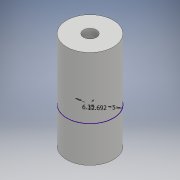
# Autodesk Inventor part: springHolder_final
Saved by Autodesk Inventor 2018 (Build 220112000, 112)
## iProperties
Created: 2017-11-09
Part Number: springHolder_final
Material: Generic
Document SubType Name: Modeling
Designer: Payal Jindal
Density: 1 g/cm^3
Appearance: Default
Author: Payal Jindal
Autodesk Inventor part; units mm, degrees
ref_plane "YZ Plane" through (0, 0, 0) normal (1, 0, 0) x (0, 1, 0)
ref_plane "XZ Plane" through (0, 0, 0) normal (0, 1, 0) x (-1, 0, 0)
ref_plane "XY Plane" through (0, 0, 0) normal (0, 0, 1) x (1, 0, 0)
sketch "Sketch1" plane through (0, 0, 0) normal (0, 0, 1) x (1, 0, 0)
  circle A0 centre (0, 0) radius 6.346
  circle A1 centre (0, 0) radius 11.346
  circle A2 centre (0, 0) radius 3.175
  dimension "d0" = 12.692
  dimension "d1" = 5
  dimension "d2" = 6.35
  constraints: 3 centre point, 3 coincident
  measures "d0" diameter of A0
  measures "d1" radial gap between concentric circles of A1 A0
  measures "d2" diameter of A2
extrude "Extrusion1" add sketch "Sketch1" against normal blind 17.7 contours A1
extrude "Extrusion2" add sketch "Sketch1" along normal blind 30 contours A0 | A1
body "Solid1"
